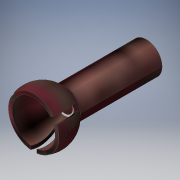
# Autodesk Inventor part: Castor New
Saved by Autodesk Inventor 2016 (Build 200138000, 138)
## iProperties
Created: 2017-09-07
Part Number: Castor New
Material: Generic
Document SubType Name: Modeling
Designer: student
Density: 1 g/cm^3
Appearance: Default
Author: student
Autodesk Inventor part; units mm, degrees
ref_plane "YZ Plane" through (0, 0, 0) normal (1, 0, 0) x (0, 1, 0)
ref_plane "XZ Plane" through (0, 0, 0) normal (0, 1, 0) x (-1, 0, 0)
ref_plane "XY Plane" through (0, 0, 0) normal (0, 0, 1) x (1, 0, 0)
sketch "Sketch1" plane through (0, 0, 0) normal (0, 0, 1) x (1, 0, 0)
  circle A0 centre (0, 0) radius 6.1169
  constraints: 1 centre point, 1 coincident
extrude "Extrusion1" add sketch "Sketch1" along normal blind 31.75
sketch "Sketch2" plane through (0, 0, 0) normal (0, 1, 0) x (-1, 0, 0)
  line L0 (0.031, 43.3682) -> (0.031, 31.8333)
  line L1 (9.8906, 43.9253) -> (8.6415, 43.9253)
  line L2 (-8.3895, 43.9713) -> (-9.7236, 43.9713)
  line L3 (6.1169, 31.75) -> (-6.1169, 31.75) projected
  line L4 (5.7447, 31.75) -> (-5.7447, 31.75)
  arc A0 (-9.7236, 43.9713) -> (-5.7447, 31.75) centre (0.1818, 40.4378) ccw
  arc A1 (5.7447, 31.75) -> (9.8906, 43.9253) centre (0.1818, 40.4378) ccw
  arc A2 (-8.3895, 43.9713) -> (-3.0546, 31.75) centre (0.1818, 40.4378) ccw
  arc A3 (3.0546, 31.75) -> (8.6415, 43.9253) centre (0.1818, 40.4378) ccw
  line L5 (0.1818, 40.4378) -> (-4.7315, 40.4378)
  circle A4 centre (0.031, 40.4378) radius 9.144 construction
  point P0 (0, 0)
  dimension "d14" = 9.271
  dimension "d15" = 18.288
  constraints: 10 end point, 8 point on circle, 6 point on line, 5 centre point, 3 horizontal, 1 coincident, 1 vertical
  measures "d14" radius of A2
  measures "d15" diameter of A4
revolve "Revolution1" add sketch "Sketch2" angle 360 about axis through (-0.031, 0, 43.3682) along (0, 0, -1)
sketch "Sketch3" plane through (-0.031, 0, 43.9253) normal (0, 0, 1) x (-1, 0, 0)
  line L0 (-0.031, 0) -> (2.8269, 0) construction
  line L1 (-0.031, 0) -> (2.6321, 0) construction
  line L2 (1.239, 10.6058) -> (-1.301, 10.6058)
  line L3 (-1.301, 10.6058) -> (-1.301, 1.4226)
  line L4 (11.1988, -5.0171) -> (1.836, 0.3886)
  line L5 (0.566, -1.8111) -> (9.9288, -7.2168)
  line L6 (9.9288, -7.2168) -> (11.1988, -5.0171)
  circle A0 centre (-0.031, 0) radius 6.1169 projected
  line L7 (-9.6642, -7.0282) -> (-0.628, -1.8111)
  line L8 (-1.898, 0.3886) -> (-10.9342, -4.8285)
  line L9 (-10.9342, -4.8285) -> (-9.6642, -7.0282)
  line L10 (1.239, 1.4226) -> (1.239, 10.6058)
  arc A1 (1.836, 0.3886) -> (1.239, 1.4226) centre (-0.031, 0) ccw
  arc A2 (-1.301, 1.4226) -> (-1.898, 0.3886) centre (-0.031, 0) ccw
  arc A3 (-0.628, -1.8111) -> (0.566, -1.8111) centre (-0.031, 0) ccw
  point P0 (-0.031, 0)
  point P1 (5.2664, -3.0585)
  point P2 (-5.1341, -2.9642)
  dimension "d6" = 2.54
  constraints: 22 end point, 6 point on circle, 3 centre point, 3 parallel, 2 horizontal, 1 coincident, 1 perpendicular, 1 vertical, 2 other
  measures "d6" distance of L2.end L2.start
extrude "Extrusion2" cut sketch "Sketch3" along normal mid plane 18.796 contours L10 A0 L3 L2 | L10 A1 L4 A0 L5 A3 L7 L8 A2 L3 | A0 L7 L9 L8 | L4 L6 L5 A0
sketch "Sketch4" plane through (0, 0, 0) normal (0, 0, -1) x (-1, 0, 0)
  circle A0 centre (0, 0) radius 1.27
  dimension "d13" = 2.54
  constraints: 1 centre point, 1 coincident
  measures "d13" diameter of A0
extrude "Extrusion3" cut sketch "Sketch4" against normal blind 15.24
body "Solid1"
